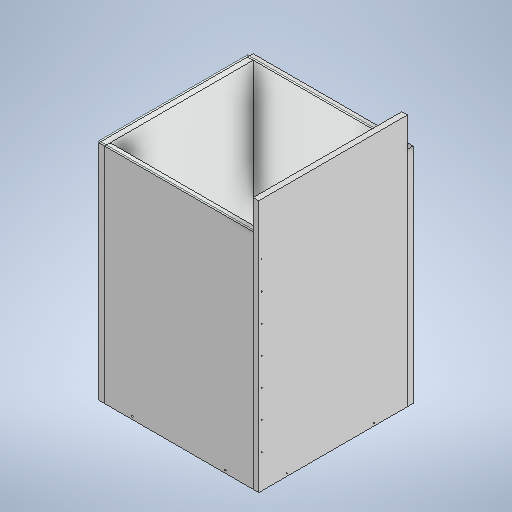
# Autodesk Inventor part: modulo1
Saved by Autodesk Inventor 2025.1 (Build 291241000, 241)
## iProperties
Created: 2024-11-02
Part Number: modulo1
Material: Genérico
Document SubType Name: Modeling
Designer: pedro
Density: 1 g/cm^3
Appearance: Padrão
Author: pedro
Autodesk Inventor part; units mm, degrees
ref_plane "YZ Plane" through (0, 0, 0) normal (1, 0, 0) x (0, 1, 0)
ref_plane "XZ Plane" through (0, 0, 0) normal (0, 1, 0) x (-1, 0, 0)
ref_plane "XY Plane" through (0, 0, 0) normal (0, 0, 1) x (1, 0, 0)
sketch "Esboço1" plane through (0, 0, 0) normal (0, 0, 1) x (1, 0, 0)
  line L0 (-200, 300) -> (200, 300)
  line L1 (200, 300) -> (200, -300)
  line L2 (200, -300) -> (-200, -300)
  line L3 (-200, -300) -> (-200, 300)
  point P0 (0, 0)
  dimension "d0" = 400
  dimension "d1" = 600
  dimension "d2" = 200
  dimension "d3" = 300
  constraints: 8 end point, 2 parallel, 1 horizontal, 1 perpendicular
  measures "d0" distance of L0.start L0.end
  measures "d1" distance of L0.end L1.end
  measures "d2" horizontal distance of point (0, 0) L0.start
  measures "d3" vertical distance of L2.end point (0, 0)
extrude "Extrusão1" add sketch "Esboço1" along normal blind 15
sketch "Esboço2" plane through (200, -300, 0) normal (1, 0, 0) x (0, 0, -1)
  line L0 (0, 0) -> (0, 600) projected
  line L1 (0, 600) -> (-15, 600) projected
  line L2 (-15, 0) -> (-15, 600) projected
  line L3 (0, 0) -> (-15, 0) projected
  line L4 (0, 0) -> (385, 0)
  line L5 (385, 0) -> (385, 600)
  line L6 (385, 600) -> (0, 600)
  line L7 (0, 600) -> (0, 0)
  point P0 (0, 300)
  dimension "d7" = 400
  constraints: 8 end point, 2 parallel, 1 horizontal, 1 perpendicular, 1 point on line
  measures "d7" distance of L5.end L1.end
extrude "Extrusão2" add sketch "Esboço2" along normal blind 15 separate body
sketch "Esboço4" plane through (200, -300, -385) normal (0, 0, -1) x (-1, 0, 0)
  line L0 (0, 0) -> (0, 600) projected
  line L1 (0, 600) -> (-15, 600) projected
  line L2 (-15, 0) -> (-15, 600) projected
  line L3 (0, 0) -> (-15, 0) projected
  line L4 (400, 0) -> (0, 0) projected
  line L5 (400, 600) -> (400, 0) projected
  line L6 (0, 600) -> (400, 600) projected
  line L7 (0, 0) -> (0, 600) projected
  point P0 (200, 300)
  point P1 (0, 600)
extrude "Extrusão4" add sketch "Esboço4" along normal blind 15 separate body
sketch "Esboço10" plane through (-200, -300, -385) normal (-1, 0, 0) x (0, 0, -1)
  line L0 (0, 0) -> (0, -600) projected
  line L1 (0, 0) -> (15, 0) projected
  line L2 (15, 0) -> (15, -600) projected
  line L3 (0, -600) -> (15, -600) projected
  line L4 (-385, -600) -> (-385, 0) projected
  line L5 (-385, 0) -> (-400, 0) projected
  line L6 (-400, -600) -> (-400, 0) projected
  line L7 (-385, -600) -> (-400, -600) projected
  line L8 (15, -600) -> (-385, -600)
  line L9 (15, 0) -> (-385, 0)
  point P0 (-385, -300)
  constraints: 4 end point, 2 collinear
extrude "Extrusão9" add sketch "Esboço10" along normal blind 15 separate body contours L0 L8 L4 L9 | L4 L7 L6 L5
sketch "Esboço11" plane through (215, -300, 0) normal (1, 0, 0) x (0, 0, -1)
  line L0 (385, 600) -> (-15, 600) projected
  line L1 (-15, 600) -> (385, 600)
  line L2 (385, 600) -> (385, 680)
  line L3 (385, 680) -> (-15, 680)
  line L4 (-15, 680) -> (-15, 600)
  point P0 (0, 300)
  dimension "d31" = 400
  dimension "d32" = 80
  constraints: 8 end point, 2 parallel, 1 horizontal, 1 perpendicular
  measures "d31" distance of L3.end L2.end
  measures "d32" distance of L2.end L1.end
extrude "Extrusão10" add sketch "Esboço11" against normal blind 15 bodies 2
sketch "Esboço12" plane through (-200, 300, 0) normal (0, 1, 0) x (1, 0, 0)
  line L0 (400, 0) -> (0, 0) projected
  line L1 (0, 0) -> (0, -15) projected
  line L2 (400, -15) -> (0, -15) projected
  line L3 (400, 0) -> (400, -15) projected
  line L4 (400, 385) -> (400, -15)
  line L5 (0, -15) -> (0, 385) projected
  line L6 (0, 385) -> (-15, 385) projected
  line L7 (-15, -15) -> (-15, 385) projected
  line L8 (0, -15) -> (-15, -15) projected
  line L9 (0, 385) -> (415, 385) projected
  line L10 (400, 385) -> (0, 385)
  point P0 (200, 0)
  point P1 (400, 0)
  point P2 (400, 0)
  constraints: 4 end point, 1 collinear, 1 perpendicular
extrude "Extrusão11" add sketch "Esboço12" along normal blind 5 separate body
ref_plane "Plano de trabalho1" through (-200, -200, -370) normal (-1, 0, 0) x (0, 0, 1)
sketch "Esboço15" plane through (-200, -200, -370) normal (-1, 0, 0) x (0, 0, 1)
  circle A0 centre (75, -92.5) radius 1.5
  line L0 (0, 0) -> (0, 15) projected
  line L1 (370, 0) -> (370, 15) projected
  line L2 (0, 15) -> (370, 15) projected
  line L3 (-15, -100) -> (385, -100) projected
  circle A1 centre (310, -92.5) radius 1.5
  line L4 (385, -100) -> (385, 500) projected
  point P0 (370, 200)
  point P1 (0, 7.5)
  point P2 (370, 7.5)
  dimension "d37" = 3
  dimension "d38" = 75
  dimension "d67" = 7.5
  dimension "d70" = 3
  dimension "d71" = 7.5
  dimension "d72" = 75
  constraints: 2 centre point, 2 midpoint
  measures "d37" diameter of A0
  measures "d38" horizontal distance of point (0, 7.5) A0.centre
  measures "d67" distance from line of L3 A0.centre
  measures "d70" diameter of A1
  measures "d71" distance from line of L3 A1.centre
  measures "d72" distance from line of L4 A1.centre
extrude "Extrusão12" cut sketch "Esboço15" along normal mid plane 50000 bodies 4 2
sketch "Esboço16" plane through (200, -300, 0) normal (-1, 0, 0) x (0, 0, 1)
  line L0 (0, 600) -> (0, 0) projected
  line L1 (0, 0) -> (0, 600) projected
  line L2 (-385, 0) -> (-385, 600) projected
  line L3 (-385, 600) -> (-385, 0) projected
  line L4 (-385, 0) -> (-385, 680) projected
  line L5 (15, 0) -> (-385, 0) projected
  line L6 (15, 0) -> (15, 680) projected
  line L7 (15, 680) -> (-385, 680) projected
  line L8 (0, 0) -> (0, 600) projected
  line L9 (0, 600) -> (-385, 600)
  line L10 (0, 560) -> (-385, 560)
  point P0 (0, 300)
  dimension "d44" = 40
  constraints: 4 end point, 2 perpendicular, 2 point on line
  measures "d44" distance between parallel lines of L9 L10
extrude "Extrusão13" add sketch "Esboço16" along normal blind 15 separate body contours L0 L10 L2 L9
sketch "Esboço17" plane through (200, -300, -400) normal (0, 0, -1) x (-1, 0, 0)
  line L0 (400, 0) -> (0, 0) projected
  line L1 (400, 600) -> (400, 0) projected
  line L2 (0, 600) -> (400, 600) projected
  line L3 (0, 0) -> (0, 600) projected
  line L4 (400, 600) -> (400, 0) projected
  line L5 (400, 0) -> (415, 0) projected
  line L6 (415, 600) -> (415, 0) projected
  line L7 (400, 600) -> (415, 600) projected
  line L8 (400, 0) -> (400, 600) projected
  line L9 (400, 0) -> (400, 600) projected
  line L10 (400, 0) -> (400, 600) projected
  line L11 (400, 0) -> (400, 600) projected
  point P0 (200, 300)
  point P1 (400, 600)
extrude "Extrusão14" add sketch "Esboço17" against normal blind 15 contours L1 L7 L6 L5 bodies 3
sketch "Esboço18" plane through (-200, -300, 0) normal (0, -1, 0) x (1, 0, 0)
  line L0 (400, 15) -> (400, -385) projected
  line L1 (400, 15) -> (400, -385) projected
  line L2 (0, 0) -> (400, 0) projected
  line L3 (400, 0) -> (0, 0) projected
  line L4 (0, -385) -> (0, 15) projected
  line L5 (0, 15) -> (0, -385) projected
  line L6 (0, -385) -> (400, -385)
  line L7 (415, -385) -> (-15, -385) projected
  point P0 (200, 0)
  point P1 (0, -385)
  constraints: 2 end point, 1 collinear
extrude "Extrusão15" add sketch "Esboço18" against normal blind 15 separate body
sketch "Esboço19" plane through (0, 0, 15) normal (0, 0, 1) x (1, 0, 0)
  circle A0 centre (-125, -292.5) radius 2
  line L0 (-200, -300) -> (-200, 300) projected
  line L1 (-200, -300) -> (200, -300) projected
  circle A1 centre (125, -292.5) radius 2
  line L2 (200, -300) -> (200, 380) projected
  point P0 (0, 0)
  dimension "d51" = 4
  dimension "d52" = 75
  dimension "d53" = 7.5
  dimension "d54" = 4
  dimension "d55" = 75
  dimension "d66" = 7.5
  constraints: 2 centre point
  measures "d51" diameter of A0
  measures "d52" distance from line of L0 A0.centre
  measures "d53" distance from line of L1 A0.centre
  measures "d54" diameter of A1
  measures "d55" distance from line of L2 A1.centre
  measures "d66" distance from line of L1 A1.centre
extrude "Extrusão16" cut sketch "Esboço19" along normal mid plane 5000 bodies 1 3
sketch "Esboço20" plane through (185, -300, 0) normal (-1, 0, 0) x (0, 0, 1)
  circle A0 centre (-310, 580) radius 2
  line L0 (-385, 600) -> (-385, 560) projected
  line L1 (0, 600) -> (-385, 600) projected
  circle A1 centre (-75, 580) radius 2
  line L2 (0, 560) -> (0, 600) projected
  point P0 (0, 300)
  point P1 (0, 580)
  dimension "d58" = 4
  dimension "d59" = 75
  dimension "d60" = 20
  dimension "d61" = 4
  dimension "d62" = 75
  dimension "d63" = 20
  constraints: 2 centre point, 1 midpoint
  measures "d58" diameter of A0
  measures "d59" distance from line of L0 A0.centre
  measures "d60" distance from line of L1 A0.centre
  measures "d61" diameter of A1
  measures "d62" distance of point (0, 580) A1.centre
  measures "d63" distance from line of L1 A1.centre
extrude "Extrusão17" cut sketch "Esboço20" against normal blind 5000 bodies 6
sketch "Esboço22" plane through (-215, -300, -385) normal (-1, 0, 0) x (0, 0, 1)
  circle A0 centre (392.5, 90) radius 1.5
  line L0 (400, 0) -> (400, 600) projected
  circle A1 centre (392.5, 165) radius 1.5
  circle A2 centre (392.5, 240) radius 1.5
  circle A3 centre (392.5, 315) radius 1.5
  circle A4 centre (392.5, 390) radius 1.5
  circle A5 centre (392.5, 465) radius 1.5
  circle A6 centre (392.5, 540) radius 1.5
  point P0 (385, 300)
  point P1 (385, 15)
  dimension "d82" = 3
  dimension "d83" = 75
  dimension "d84" = 7.5
  dimension "d85" = 3
  dimension "d86" = 75
  dimension "d87" = 3
  dimension "d88" = 75
  dimension "d89" = 3
  dimension "d90" = 75
  dimension "d91" = 3
  dimension "d92" = 75
  dimension "d93" = 3
  dimension "d94" = 75
  dimension "d95" = 3
  dimension "d96" = 75
  constraints: 7 centre point
  measures "d82" diameter of A0
  measures "d83" vertical distance of point (385, 15) A0.centre
  measures "d84" distance from line of L0 A0.centre
  measures "d85" diameter of A1
  measures "d86" distance of A0.centre A1.centre
  measures "d87" diameter of A2
  measures "d88" distance of A1.centre A2.centre
  measures "d89" diameter of A3
  measures "d90" distance of A2.centre A3.centre
  measures "d91" diameter of A4
  measures "d92" distance of A3.centre A4.centre
  measures "d93" diameter of A5
  measures "d94" distance of A4.centre A5.centre
  measures "d95" diameter of A6
  measures "d96" distance of A5.centre A6.centre
extrude "Extrusão18" cut sketch "Esboço22" along normal mid plane 50000 bodies 2 4
equation "\"d2\" = 0.5 * d0"
equation "\"d3\" = 0.5 * d1"
